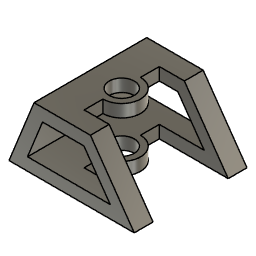
practice_2 v2 (Autodesk Fusion 360 design; units mm, degrees)
Autodesk Fusion 360 part; units mm, degrees
note: some values were not read from the file. Set by a fixed rule: which face or edge a step refers to.
sketch "Sketch2" plane through (0, 0, 0) normal (0, 1, 0) x (1, 0, 0)
  line L0 (0, 0) -> (100, 0)
  line L1 (100, 0) -> (100, -50)
  line L2 (100, -50) -> (0, -50)
  line L3 (0, -50) -> (0, 0)
  dimension "d3" = 100
  dimension "d4" = 50
  constraint horizontal L0
  constraint vertical L1
  constraint horizontal L2
  constraint vertical L3
  constraint coincident L0.start L3.end
  measures "d3" distance of L0.start L0.end
  measures "d4" distance of L0.start L2.end
extrude "Extrude1" add sketch "Sketch2" along normal blind 90
chamfer "Chamfer1" distance 35 distance2 50 1 edges at (100, 45, 50) measured on face at (66.6667, 30, 50)
chamfer "Chamfer2" distance 50 distance2 20 1 edges at (0, 45, 50) measured on face at (0, 30, 33.3333)
shell "Shell1" thickness 10 removed faces 1 at (55.0023, 0, 16.6733)
extrude "Extrude2" cut 1 faces at (51.7891, 80, 20) along direction (0, 1, 0) blind 70
sketch "Sketch5" plane through (0, 0, 0) normal (0, 0, -1) x (1, 0, 0)
  line L0 (100, 0) -> (0, 0)
  line L1 (0, 0) -> (0, -90)
  line L2 (0, -90) -> (100, -90)
  line L3 (100, -90) -> (100, 0)
  line L4 (100, -75) -> (100, -15)
  line L5 (100, -15) -> (45, -15)
  line L6 (45, -15) -> (45, -75)
  line L7 (45, -75) -> (100, -75)
  line L8 (100, -75) -> (100, -15)
  point P0 (100, -15)
  point P1 (100, -75)
  dimension "d43" = 55
  dimension "d44" = 60
  constraint coincident L3 P0
  constraint coincident L3 P1
  constraint vertical L4
  constraint coincident P0 L4.end
  constraint horizontal L5
  constraint vertical L6
  constraint horizontal L7
  constraint vertical L8
  measures "d43" distance of P0 L5.end
  measures "d44" distance of P0 P1
extrude "Extrude12" cut sketch "Sketch5" against normal blind 180 contours L3 L4 L5 L6 L7 L8
sketch "Sketch9" plane through (0, 0, 50) normal (0, 0, 1) x (-1, 0, 0)
  line L0 (-45, -75) -> (-65, -75)
  line L1 (-65, -75) -> (-65, -90)
  line L2 (-65, -90) -> (-20, -90)
  line L3 (-20, -90) -> (-20, 0)
  line L4 (-20, 0) -> (-65, 0)
  line L5 (-65, 0) -> (-65, -15)
  line L6 (-65, -15) -> (-45, -15)
  line L7 (-45, -15) -> (-45, -75)
  circle A0 centre (-45, -45) radius 15
  circle A1 centre (-45, -45) radius 10
  point P0 (-45, -90)
  point P1 (-45, 0)
  point P2 (-45, -45)
  dimension "d47" = 30
  dimension "d48" = 20
  constraint coincident L2 P0
  constraint coincident L4 P1
  constraint midpoint L7 P2
  constraint coincident P2 A0.centre
  measures "d47" diameter of A0
  measures "d48" diameter of A1
sketch "Sketch10" plane through (0, 0, 0) normal (0, 0, -1) x (1, 0, 0)
  circle A0 centre (45, -45) radius 10
  circle A1 centre (45, -45) radius 15
  dimension "d49" = 20
  dimension "d50" = 30
  constraint concentric A0 A1
  measures "d49" diameter of A0
  measures "d50" diameter of A1
extrude "Extrude13" cut sketch "Sketch10" against normal blind 11 contours A0
extrude "Extrude14" add sketch "Sketch10" against normal blind 10
extrude "Extrude15" cut sketch "Sketch9" against normal blind 11 contours L7 A1 | L7 A1
extrude "Extrude16" add sketch "Sketch9" against normal blind 10 contours L7 A0 A1 picked at (-51.4323, -56.6393)
extrude "Extrude10" [suppressed]
sketch "Sketch8" plane through (0, 0, 50) normal (0, 0, 1) x (-1, 0, 0)
  line L0 (-50, -75) -> (-65, -75)
  line L1 (-65, -75) -> (-65, -90)
  line L2 (-65, -90) -> (-20, -90)
  line L3 (-20, -90) -> (-20, 0)
  line L4 (-20, 0) -> (-65, 0)
  line L5 (-65, 0) -> (-65, -15)
  line L6 (-65, -15) -> (-50, -15)
  line L7 (-50, -15) -> (-50, -75)
sketch "Sketch6" plane through (0, 0, 50) normal (0, 0, 1) x (-1, 0, 0)
  line L0 (-50, -75) -> (-65, -75)
  line L1 (-65, -75) -> (-65, -90)
  line L2 (-65, -90) -> (-20, -90)
  line L3 (-20, -90) -> (-20, 0)
  line L4 (-20, 0) -> (-65, 0)
  line L5 (-65, 0) -> (-65, -15)
  line L6 (-65, -15) -> (-50, -15)
  line L7 (-50, -15) -> (-50, -75)
  circle A0 centre (-42.5, -40) radius 15
  point P0 (-42.5, -90)
  point P1 (-42.5, 0)
  point P2 (-50, -45)
  point P3 (-42.5, -45)
  point P4 (-42.5, -40)
  dimension "d38" = 30
  constraint midpoint L2 P0
  constraint midpoint L4 P1
  constraint midpoint L7 P2
  constraint coincident P4 A0.centre
  measures "d38" diameter of A0
extrude "Extrude11" [suppressed]
sketch "Sketch3" plane through (0, 0, 50) normal (0, 0, 1) x (-1, 0, 0)
  line L0 (-20, -90) -> (-20, 0)
  line L1 (-20, 0) -> (-65, 0)
  line L2 (-65, 0) -> (-65, -90)
  line L3 (-65, -90) -> (-20, -90)
  circle A0 centre (-42.5, -39.9983) radius 15
  circle A1 centre (-42.5, -39.9983) radius 10
  line L4 (-65, 0) -> (-65, -15)
  line L5 (-65, -90) -> (-65, -75)
  line L6 (-65, -15) -> (-42.5, -15)
  line L7 (-42.5, -15) -> (-42.5, -75)
  line L8 (-42.5, -75) -> (-65, -75)
  line L9 (-65, -75) -> (-65, -15)
  point P0 (-42.5, -90)
  point P1 (-42.5, -18.8599)
  point P2 (-42.5, 0)
  point P3 (-65, -45)
  point P4 (-20, -45)
  point P5 (-42.5, -44.9983)
  point P6 (-42.5, -44.9983)
  point P7 (-42.5, -39.9983)
  dimension "d16" = 30
  dimension "d17" = 20
  dimension "d18" = 15
  dimension "d19" = 60
  constraint midpoint L3 P0
  constraint midpoint L1 P2
  constraint midpoint L2 P3
  constraint midpoint L0 P4
  constraint coincident P7 A0.centre
  constraint concentric A0 A1
  constraint coincident L1.end L2.start
  constraint coincident L2 L4.end
  constraint coincident L2.end L3.start
  constraint coincident L2 L5.end
  constraint perpendicular L3 L5
  constraint horizontal L6
  constraint vertical L7
  constraint horizontal L8
  constraint vertical L9
  measures "d16" diameter of A0
  measures "d17" diameter of A1
  measures "d18" distance of L1.end L4.end
  measures "d19" distance of L4.end L5.end
extrude "Extrude3" [suppressed]
extrude "Extrude4" [suppressed]
sketch "Sketch4" plane through (67.1141, 0, 46.9799) normal (0.819232, 0, 0.573462) x (0, 1, 0)
  line L0 (90, -57.3462) -> (90, 3.6865)
  line L1 (90, 3.6865) -> (0, 3.6865)
  line L2 (0, 3.6865) -> (0, -57.3462)
  line L3 (0, -57.3462) -> (90, -57.3462)
  line L4 (14.9899, 3.6865) -> (74.9899, 3.6865)
  line L5 (74.9899, 3.6865) -> (74.9899, -57.3951)
  line L6 (74.9899, -57.3951) -> (14.9899, -57.3951)
  line L7 (14.9899, -57.3951) -> (14.9899, 3.6865)
  point P0 (74.9998, 3.6865)
  point P1 (14.9899, 3.6865)
  point P2 (14.9999, 3.6865)
  dimension "d27" = 60
  constraint coincident L1 P0
  constraint coincident L1 P1
  constraint coincident L1 P2
  constraint horizontal L4
  constraint vertical L5
  constraint horizontal L6
  constraint vertical L7
  constraint coincident P1 L4.start
  measures "d27" distance of P1 L4.end
ref_plane "WorkPlane1" through (65, 45, 50) normal (1, 0, 0) x (0, -1, 0)
extrude "Extrude5" [suppressed]
extrude "Extrude6" [suppressed]
extrude "Extrude7" [suppressed]
extrude "Extrude8" [suppressed]
extrude "Extrude9" [suppressed]
